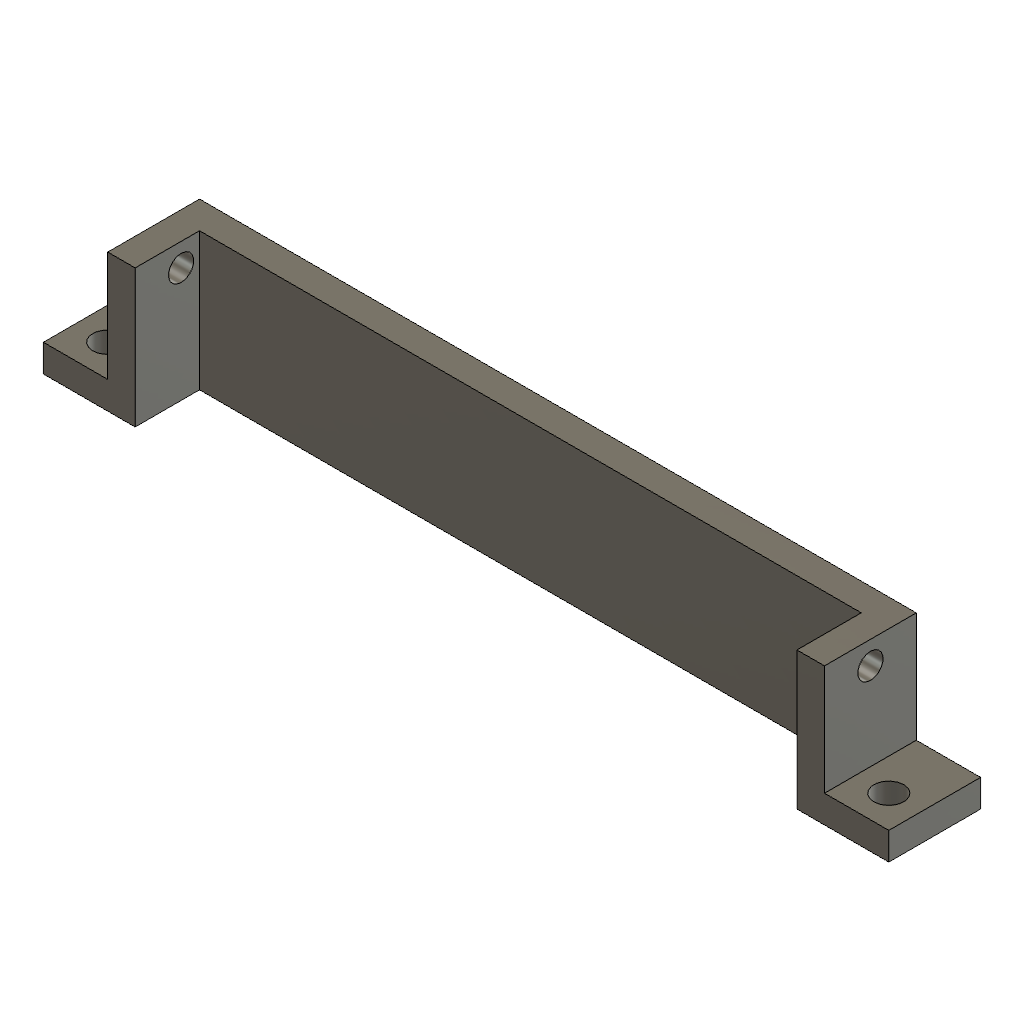
TankBot Phone Base (Autodesk Fusion 360 design; units mm, degrees)
Autodesk Fusion 360 part; units mm, degrees
box "BoxPrimitive1" add length 3 width 78 height 10 placed x (0, 0, 1) y (1, 0, 0) z (0, 1, 0) at (0, 0, 0)
box "BoxPrimitive2" add length 10 width 3 height 7 placed x (0, -1, 0) y (1, 0, 0) z (0, 0, 1) at (75, 10, 3)
box "BoxPrimitive3" add length 3 width 10 height 6 placed x (0, 1, 0) y (0, 0, 1) z (1, 0, 0) at (78, 0, 0)
box "BoxPrimitive4" add length 10 width 3 height 7 placed x (0, -1, 0) y (1, 0, 0) z (0, 0, 1) at (0, 10, 3)
box "BoxPrimitive5" add length 3 width 10 height -6 placed x (0, -1, 0) y (0, 0, -1) z (1, 0, 0) at (0, 3, 10)
extrude "Extrude1" add 1 faces at (84, 1, 6.6667) along direction (1, 0, 0) blind 1
extrude "Extrude2" add 1 faces at (-6, 2, 3.3333) along direction (-1, 0, 0) blind 1
hole "Hole3" at (-3.5, 3, 6.5) direction (0, -1, 0) diameter 3.25 depth 3 tip angle 180
hole "Hole4" at (81.5, 3, 6.5) direction (0, -1, 0) diameter 3.25 depth 3 tip angle 180
extrude "Extrude3" add 1 faces at (27, 10, 1) along direction (0, 1, 0) blind 5
hole "Hole5" at (0, 12.5, 5) direction (1, 0, 0) diameter 2.75 depth 160 tip angle 180
